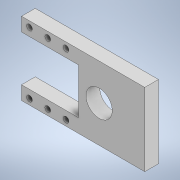
# Autodesk Inventor part: Sopoter_gripperM
Saved by Autodesk Inventor 2021.4 (Build 254397000, 397)
## iProperties
Created: 2022-02-03
Part Number: Sopoter_gripperM
Material: Genérico
Document SubType Name: Modeling
Designer: epm01
Density: 1 g/cm^3
Appearance: Valor por defecto
Author: epm01
Autodesk Inventor part; units mm, degrees
ref_plane "YZ Plane" through (0, 0, 0) normal (1, 0, 0) x (0, 1, 0)
ref_plane "XZ Plane" through (0, 0, 0) normal (0, 1, 0) x (-1, 0, 0)
ref_plane "XY Plane" through (0, 0, 0) normal (0, 0, 1) x (1, 0, 0)
sketch "Boceto1" plane through (0, 0, 0) normal (0, 0, 1) x (1, 0, 0)
  line L0 (0, 0) -> (0, 16)
  line L1 (0, 16) -> (-54, 16)
  line L2 (-54, 16) -> (-54, 10)
  line L3 (-54, 10) -> (-29, 10)
  line L4 (0, 0) -> (-39.6047, 0)
  line L5 (-29, 10) -> (-29, 0)
  line L6 (-54, 13.5) -> (-50.5, 13.5)
  line L7 (-50.5, 13.5) -> (-50.5, 10)
  circle A0 centre (-50.5, 13.5) radius 1.25
  line L8 (-50.5, 13.5) -> (-42.5, 13.5)
  line L9 (-42.5, 13.5) -> (-34.5, 13.5)
  circle A1 centre (-42.5, 13.5) radius 1.25
  circle A2 centre (-34.5, 13.5) radius 1.25
  line L10 (0, 0) -> (0, -16)
  line L11 (0, -16) -> (-54, -16)
  line L12 (-54, -16) -> (-54, -10)
  line L13 (-54, -10) -> (-29, -10)
  line L14 (-29, -10) -> (-29, 0)
  circle A3 centre (-50.5, -13.5) radius 1.25
  circle A4 centre (-42.5, -13.5) radius 1.25
  circle A5 centre (-34.5, -13.5) radius 1.25
  point P0 (-54, -13.5)
  point P1 (-50.5, 12.25)
  point P2 (-51.75, 13.5)
  dimension "d0" = 10
  dimension "d1" = 25
  dimension "d2" = 6
  dimension "d3" = 54
  dimension "d4" = 3.5
  dimension "d5" = 3.5
  dimension "d6" = 2.5
  dimension "d7" = 8
  dimension "d8" = 8
  dimension "d9" = 2.5
  dimension "d10" = 2.5
  constraints: 30 end point, 8 symmetric about line, 6 centre point, 5 point on line, 4 perpendicular, 3 coincident, 3 horizontal, 2 vertical, 3 other
  measures "d0" distance of L3.end L5.end
  measures "d1" distance of L2.end L3.end
  measures "d2" distance of L1.end L2.end
  measures "d3" distance of L0.end L1.end
  measures "d4" distance of L6.end L7.end
  measures "d5" distance of L6.start L6.end
  measures "d6" diameter of A0
  measures "d7" distance of L8.start L8.end
  measures "d8" distance of L8.end L9.end
  measures "d9" diameter of A1
  measures "d10" diameter of A2
extrude "Extrusión1" add sketch "Boceto1" along normal blind 6 contours L4 L5 L3 L7 A0 L6 L2 L1 L0 | L10 L11 L12 L13 L14 L4 | L6 A0 L7 L3 L2
sketch "Boceto2" plane through (0, 0, 6) normal (0, 0, 1) x (1, 0, 0)
  circle A0 centre (-50.5, 13.5) radius 1.25 projected
  line L0 (-50.5, 13.5) -> (-20, 13.5)
  line L1 (-54, 10) -> (-29, 10) projected
  line L2 (-20, 13.5) -> (-20, 0)
  point P0 (0, 0)
  dimension "d13" = 30.5
  constraints: 4 end point, 1 parallel, 1 perpendicular
  measures "d13" distance of L0.start L0.end
hole "Agujero1" at (-20, 0, 6) direction (0, 0, -1) diameter 11.5 end through all
